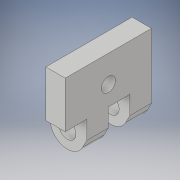
# Autodesk Inventor part: item_scharnier_teil
Saved by Autodesk Inventor 2018 (Build 220112000, 112)
## iProperties
Created: 2020-04-19
Part Number: item_scharnier_teil
Material: Generisch
Document SubType Name: Modeling
Designer: wepet
Density: 1 g/cm^3
Appearance: Vorgabe
Author: wepet
Autodesk Inventor part; units mm, degrees
ref_plane "YZ Plane" through (0, 0, 0) normal (1, 0, 0) x (0, 1, 0)
ref_plane "XZ Plane" through (0, 0, 0) normal (0, 1, 0) x (-1, 0, 0)
ref_plane "XY Plane" through (0, 0, 0) normal (0, 0, 1) x (1, 0, 0)
sketch "Skizze1" plane through (0, 0, 0) normal (0, 1, 0) x (-1, 0, 0)
  line L0 (0, 0) -> (0.9, 0)
  line L1 (0.9, 0) -> (0.9, -3)
  line L2 (0.9, -3) -> (0, -3) construction
  line L3 (0, -3) -> (0, 0)
  circle A0 centre (0.9, -3) radius 0.4
  arc A1 (0.1889, -3.3665) -> (0.9, -2.2) centre (0.9, -3) ccw
  line L4 (0, -3) -> (0.1889, -3.3665)
  dimension "d0" = 0.9
  dimension "d2" = 0.8
  dimension "d3" = 1.6
  dimension "d4" = 3
  constraints: 10 end point, 2 centre point, 2 parallel, 2 point on circle, 1 coincident, 1 horizontal, 1 perpendicular, 1 point on line, 1 tangent
  measures "d0" distance of L1.end L2.end
  measures "d2" diameter of A0
  measures "d3" diameter of A1
  measures "d4" distance of L2.end L0.start
extrude "Extrusion1" add sketch "Skizze1" along normal blind 4
sketch "Skizze2" plane through (0, 0, 0) normal (1, 0, 0) x (0, 0, -1)
  line L0 (3, 0) -> (0, 0) construction
  line L1 (3, 0) -> (3, 4) construction
  line L2 (0, 4) -> (3, 4) construction
  line L3 (0, 0) -> (0, 4) construction
  line L4 (0, 4) -> (3, 4) construction
  line L5 (2.15, 4) -> (2.15, 0) construction
  line L6 (2.15, 0) -> (4.15, 0)
  line L7 (4.15, 0) -> (4.15, 1)
  line L8 (4.15, 1) -> (2.15, 1)
  line L9 (2.15, 1) -> (2.15, 0)
  line L10 (2.15, 3) -> (4.15, 3)
  line L11 (4.15, 3) -> (4.15, 2)
  line L12 (4.15, 2) -> (2.15, 2)
  line L13 (2.15, 2) -> (2.15, 3)
  dimension "d7" = 0.85
  dimension "d8" = 2
  dimension "d9" = 1
  dimension "d10" = 1
  dimension "d11" = 1
  constraints: 18 end point, 4 parallel, 4 point on line, 3 perpendicular, 2 horizontal
  measures "d7" distance between parallel lines of L1 L5
  measures "d8" distance of L8.end L7.end
  measures "d9" distance of L6.end L7.end
  measures "d10" distance of L10.end L11.end
  measures "d11" distance between parallel lines of L8 L12
extrude "Extrusion2" cut sketch "Skizze2" against normal blind 4
sketch "Skizze4" plane through (-0.9, 0, 0) normal (-1, 0, 0) x (0, 0, 1)
  line L0 (-2.15, 1) -> (-2.15, 0) construction
  line L1 (0, 0) -> (-2.15, 0) construction
  line L2 (0, 0) -> (0, 4) construction
  line L3 (-2.2, 4) -> (0, 4) construction
  line L4 (-2.2, 3) -> (-2.2, 4) construction
  line L5 (-2.2, 3) -> (-2.15, 3) construction
  line L6 (-2.15, 3) -> (-2.15, 2) construction
  line L7 (-2.15, 2) -> (-2.2, 2) construction
  line L8 (-2.2, 1) -> (-2.2, 2) construction
  line L9 (-2.2, 1) -> (-2.15, 1) construction
  line L10 (0, 0) -> (0, 4) construction
  line L11 (0, 2) -> (-2.15, 2) construction
  line L12 (-1.25, 4) -> (-1.25, 0) construction
  point P0 (-1.25, 2)
  dimension "d22" = 1.25
  constraints: 4 end point, 2 midpoint, 2 perpendicular, 2 point on line
  measures "d22" distance between parallel lines of L2 L12
hole "Bohrung2" at (-0.9, 2, -1.25) direction (1, 0, 0) diameter 0.65 end through all countersink diameter 1 countersink angle 90
